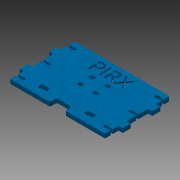
# Autodesk Inventor part: czesc5
Saved by Autodesk Inventor 2013 (Build 170138000, 138)
## iProperties
Created: 2014-01-17
Part Number: czesc5
Material: Generic
Document SubType Name: Modeling
Designer: dzban
Density: 1 g/cm^3
Author: dzban
Autodesk Inventor part; units mm, degrees
ref_plane "YZ Plane" through (0, 0, 0) normal (1, 0, 0) x (0, 1, 0)
ref_plane "XZ Plane" through (0, 0, 0) normal (0, 1, 0) x (-1, 0, 0)
ref_plane "XY Plane" through (0, 0, 0) normal (0, 0, 1) x (1, 0, 0)
sketch "Sketch1" plane through (0, 0, 0) normal (0, 0, 1) x (1, 0, 0)
  line L0 (24.6928, -26.0637) -> (24.6928, -36.0637)
  line L1 (24.6928, -36.0637) -> (83.1928, -36.0637)
  line L2 (83.1928, -36.0637) -> (83.1928, -27.5637)
  line L3 (83.1928, -27.5637) -> (76.1894, -27.5637)
  line L4 (76.1894, -27.5637) -> (76.1894, -28.8137)
  line L5 (76.1894, -28.8137) -> (74.3894, -28.8137)
  line L6 (74.3894, -28.8137) -> (74.3894, -27.5637)
  line L7 (74.3894, -27.5637) -> (71.3894, -27.5637)
  line L8 (71.3894, -27.5637) -> (71.3894, -24.5637)
  line L9 (71.3894, -24.5637) -> (74.3894, -24.5637)
  line L10 (74.3894, -24.5637) -> (74.3894, -23.3137)
  line L11 (74.3894, -23.3137) -> (76.1894, -23.3137)
  line L12 (76.1894, -23.3137) -> (76.1894, -24.5637)
  line L13 (76.1894, -24.5637) -> (83.1928, -24.5637)
  line L14 (83.1928, -24.5637) -> (83.1928, -16.1637)
  line L15 (83.1928, -16.1637) -> (89.1928, -16.0637)
  line L16 (89.1928, -16.0637) -> (89.1928, -4.2637)
  line L17 (89.1928, -4.2637) -> (83.1928, -4.1637)
  line L18 (83.1928, -4.1637) -> (83.1928, 9.9363)
  line L19 (83.1928, 9.9363) -> (76.1894, 9.9363)
  line L20 (76.1894, 9.9363) -> (76.1894, 8.6863)
  line L21 (76.1894, 8.6863) -> (74.3894, 8.6863)
  line L22 (74.3894, 8.6863) -> (74.3894, 9.9363)
  line L23 (74.3894, 9.9363) -> (71.3894, 9.9363)
  line L24 (71.3894, 9.9363) -> (71.3894, 12.9363)
  line L25 (71.3894, 12.9363) -> (74.3894, 12.9363)
  line L26 (74.3894, 12.9363) -> (74.3894, 14.1863)
  line L27 (74.3894, 14.1863) -> (76.1894, 14.1863)
  line L28 (76.1894, 14.1863) -> (76.1894, 12.9363)
  line L29 (76.1894, 12.9363) -> (83.1928, 12.9363)
  line L30 (83.1928, 12.9363) -> (83.1928, 27.0363)
  line L31 (83.1928, 27.0363) -> (89.1928, 27.1363)
  line L32 (89.1928, 27.1363) -> (89.1928, 38.9363)
  line L33 (89.1928, 38.9363) -> (83.1928, 39.0363)
  line L34 (83.1928, 39.0363) -> (83.1928, 47.4363)
  line L35 (83.1928, 47.4363) -> (76.1894, 47.4363)
  line L36 (76.1894, 47.4363) -> (76.1894, 46.1863)
  line L37 (76.1894, 46.1863) -> (74.3894, 46.1863)
  line L38 (74.3894, 46.1863) -> (74.3894, 47.4363)
  line L39 (74.3894, 47.4363) -> (71.3894, 47.4363)
  line L40 (71.3894, 47.4363) -> (71.3894, 50.4363)
  line L41 (71.3894, 50.4363) -> (74.3894, 50.4363)
  line L42 (74.3894, 50.4363) -> (74.3894, 51.6863)
  line L43 (74.3894, 51.6863) -> (76.1894, 51.6863)
  line L44 (76.1894, 51.6863) -> (76.1894, 50.4363)
  line L45 (76.1894, 50.4363) -> (83.1928, 50.4363)
  line L46 (83.1928, 50.4363) -> (83.1928, 52.9373)
  line L47 (83.1928, 55.937) -> (83.1928, 56.9363)
  arc A0 (83.1928, 56.9363) -> (81.1928, 58.9363) centre (81.1928, 56.9363) ccw
  line L48 (81.1928, 58.9363) -> (-53.8072, 58.9363)
  arc A1 (-53.8072, 58.9363) -> (-55.8072, 56.9363) centre (-53.8072, 56.9363) ccw
  line L49 (-55.8072, 56.9363) -> (-55.8072, 55.9363)
  line L50 (-55.8072, 52.9363) -> (-55.8072, 50.4363)
  line L51 (-55.8072, 50.4363) -> (-48.8072, 50.4363)
  line L52 (-48.8072, 50.4363) -> (-48.8072, 51.6863)
  line L53 (-48.8072, 51.6863) -> (-47.0072, 51.6863)
  line L54 (-47.0072, 51.6863) -> (-47.0072, 50.4363)
  line L55 (-47.0072, 50.4363) -> (-44.0716, 50.4363)
  line L56 (-44.0716, 50.4363) -> (-44.0716, 47.4363)
  line L57 (-44.0716, 47.4363) -> (-47.0072, 47.4363)
  line L58 (-47.0072, 47.4363) -> (-47.0072, 46.1863)
  line L59 (-47.0072, 46.1863) -> (-48.8072, 46.1863)
  line L60 (-48.8072, 46.1863) -> (-48.8072, 47.4363)
  line L61 (-48.8072, 47.4363) -> (-55.8072, 47.4363)
  line L62 (-55.8072, 47.4363) -> (-55.8072, 39.0363)
  line L63 (-55.8072, 39.0363) -> (-61.8072, 38.9363)
  line L64 (-61.8072, 38.9363) -> (-61.8072, 27.1363)
  line L65 (-61.8072, 27.1363) -> (-55.8072, 27.0363)
  line L66 (-55.8072, 27.0363) -> (-55.8072, 12.9363)
  line L67 (-55.8072, 12.9363) -> (-48.8072, 12.9363)
  line L68 (-48.8072, 12.9363) -> (-48.8072, 14.1863)
  line L69 (-48.8072, 14.1863) -> (-47.0072, 14.1863)
  line L70 (-47.0072, 14.1863) -> (-47.0072, 12.9363)
  line L71 (-47.0072, 12.9363) -> (-44.0716, 12.9363)
  line L72 (-44.0716, 12.9363) -> (-44.0716, 9.9363)
  line L73 (-44.0716, 9.9363) -> (-47.0072, 9.9363)
  line L74 (-47.0072, 9.9363) -> (-47.0072, 8.6863)
  line L75 (-47.0072, 8.6863) -> (-48.8072, 8.6863)
  line L76 (-48.8072, 8.6863) -> (-48.8072, 9.9363)
  line L77 (-48.8072, 9.9363) -> (-55.8072, 9.9363)
  line L78 (-55.8072, 9.9363) -> (-55.8072, -4.1637)
  line L79 (-55.8072, -4.1637) -> (-61.8072, -4.2637)
  line L80 (-61.8072, -4.2637) -> (-61.8072, -16.0637)
  line L81 (-61.8072, -16.0637) -> (-55.8072, -16.1637)
  line L82 (-55.8072, -16.1637) -> (-55.8072, -24.5637)
  line L83 (-55.8072, -24.5637) -> (-48.8072, -24.5637)
  line L84 (-48.8072, -24.5637) -> (-48.8072, -23.3137)
  line L85 (-48.8072, -23.3137) -> (-47.0072, -23.3137)
  line L86 (-47.0072, -23.3137) -> (-47.0072, -24.5637)
  line L87 (-47.0072, -24.5637) -> (-44.0716, -24.5637)
  line L88 (-44.0716, -24.5637) -> (-44.0716, -27.5637)
  line L89 (-44.0716, -27.5637) -> (-47.0072, -27.5637)
  line L90 (-47.0072, -27.5637) -> (-47.0072, -28.8137)
  line L91 (-47.0072, -28.8137) -> (-48.8072, -28.8137)
  line L92 (-48.8072, -28.8137) -> (-48.8072, -27.5637)
  line L93 (-48.8072, -27.5637) -> (-55.8072, -27.5637)
  line L94 (-55.8072, -27.5637) -> (-55.8072, -36.0637)
  line L95 (-55.8072, -36.0637) -> (2.6928, -36.0637)
  line L96 (2.6928, -36.0637) -> (2.6928, -26.0637)
  line L97 (2.6928, -26.0637) -> (24.6928, -26.0637)
  line L98 (53.2575, -19.0636) -> (53.2575, -25.4636)
  line L99 (53.2575, -25.4636) -> (41.4575, -25.4636)
  line L100 (41.4575, -25.4636) -> (41.4575, -19.0636)
  line L101 (41.4575, -19.0636) -> (53.2575, -19.0636)
  line L102 (-13.9425, -19.0636) -> (-13.9425, -25.4636)
  line L103 (-13.9425, -25.4636) -> (-25.7425, -25.4636)
  line L104 (-25.7425, -25.4636) -> (-25.7425, -19.0636)
  line L105 (-25.7425, -19.0636) -> (-13.9425, -19.0636)
  line L106 (5.6928, 6.2364) -> (-0.7072, 6.2364)
  line L107 (-0.7072, 6.2364) -> (-0.7072, 11.2364)
  line L108 (-0.7072, 11.2364) -> (5.6928, 11.2364)
  line L109 (5.6928, 11.2364) -> (5.6928, 6.2364)
  line L110 (28.0928, 6.2364) -> (21.6928, 6.2364)
  line L111 (21.6928, 6.2364) -> (21.6928, 11.2364)
  line L112 (21.6928, 11.2364) -> (28.0928, 11.2364)
  line L113 (28.0928, 11.2364) -> (28.0928, 6.2364)
  line L114 (28.0928, 23.8364) -> (21.6928, 23.8364)
  line L115 (21.6928, 23.8364) -> (21.6928, 28.8364)
  line L116 (21.6928, 28.8364) -> (28.0928, 28.8364)
  line L117 (28.0928, 28.8364) -> (28.0928, 23.8364)
  line L118 (5.6928, 28.8364) -> (5.6928, 23.8364)
  line L119 (5.6928, 23.8364) -> (-0.7072, 23.8364)
  line L120 (-0.7072, 23.8364) -> (-0.7072, 28.8364)
  line L121 (-0.7072, 28.8364) -> (5.6928, 28.8364)
  line L122 (-55.8072, 52.9363) -> (-55.8072, 55.9363)
  line L123 (83.1928, 52.9373) -> (83.1928, 55.937)
  point P0 (0, 0)
  dimension "d0" = 58.9363
  dimension "d2" = 139
  dimension "d3" = 95
  dimension "d4" = 55.8072
  dimension "d5" = 6
  dimension "d6" = 2
  dimension "d7" = 12
  dimension "d8" = 12
  dimension "d9" = 11.7356
  dimension "d10" = 2.9356
  dimension "d11" = 1.8
  dimension "d12" = 3
  dimension "d13" = 1.25
  dimension "d14" = 1.25
  dimension "d15" = 8.5
  dimension "d16" = 3
  dimension "d17" = 1.25
  dimension "d18" = 1.25
  dimension "d19" = 8.5
  dimension "d20" = 19.9
  dimension "d21" = 0.1
  dimension "d22" = 11.8
  dimension "d23" = 46
  dimension "d24" = 3
  dimension "d25" = 1.25
  dimension "d26" = 1.25
  dimension "d27" = 19.9
  dimension "d28" = 6.4
  dimension "d29" = 5
  dimension "d30" = 6.4
  dimension "d31" = 5
  dimension "d32" = 12.6
  dimension "d33" = 16
  dimension "d34" = 30.1
  dimension "d35" = 55.1
  dimension "d36" = 11.8033
  dimension "d37" = 3
  dimension "d38" = 1.8
  dimension "d39" = 6
  dimension "d40" = 22
  dimension "d41" = 10
  dimension "d42" = 58.5
  constraints: 248 end point, 88 parallel, 65 collinear, 24 perpendicular, 16 tangent, 4 horizontal alignment, 4 point on circle, 2 centre point, 1 equal radius, 1 horizontal
  measures "d0" distance from line of L48 point (0, 0)
  measures "d2" distance between parallel lines of L47 L49
  measures "d3" distance between parallel lines of L48 L95
  measures "d4" distance from line of L49 point (0, 0)
  measures "d5" distance between parallel lines of L94 L80
  measures "d6" radius of A1
  measures "d7" distance of L62.end L65.end
  measures "d8" distance of L78.end L81.end
  measures "d9" distance between parallel lines of L50 L56
  measures "d10" distance between parallel lines of L56 L54
  measures "d11" distance between parallel lines of L54 L52
  measures "d12" distance between parallel lines of L51 L61
  measures "d13" distance between parallel lines of L53 L51
  measures "d14" distance from line of L57 L58.end
  measures "d15" distance between parallel lines of L48 L51
  measures "d16" distance between parallel lines of L83 L93
  measures "d17" distance between parallel lines of L89 L91
  measures "d18" distance between parallel lines of L85 L87
  measures "d19" distance between parallel lines of L93 L95
  measures "d20" distance from line of L48 L62.end
  measures "d21" vertical distance of L62.end L63.end
  measures "d22" distance of L63.end L64.end
  measures "d23" distance between parallel lines of L77 L95
  measures "d24" distance between parallel lines of L67 L77
  measures "d25" distance between parallel lines of L73 L75
  measures "d26" distance between parallel lines of L71 L69
  measures "d27" distance from line of L81.end L95
  measures "d28" distance between parallel lines of L118 L120
  measures "d29" distance between parallel lines of L121 L119
  measures "d30" distance between parallel lines of L117 L115
  measures "d31" distance between parallel lines of L108 L106
  measures "d32" distance between parallel lines of L119 L108
  measures "d33" distance between parallel lines of L115 L118
  measures "d34" distance between parallel lines of L48 L121
  measures "d35" distance between parallel lines of L120 L66
  measures "d36" distance between parallel lines of L46 L40
  measures "d37" distance between parallel lines of L42 L40
  measures "d38" distance between parallel lines of L44 L42
  measures "d39" distance from line of L47.start L32
  measures "d40" distance between parallel lines of L0 L96
  measures "d41" distance between parallel lines of L97 L1
  measures "d42" distance between parallel lines of L96 L94
extrude "Extrusion1" add sketch "Sketch1" along normal blind 6
fillet "Fillet1" radius 2 4 edges at (2.6928, -36.0637, 3) (2.6928, -26.0637, 3) (24.6928, -26.0637, 3) (24.6928, -36.0637, 3)
sketch "Sketch9" plane through (0, 0, 6) normal (0, 0, 1) x (1, 0, 0)
  line L0 (-15.0286, 52.3696) -> (-4.2568, 52.3696) construction
  line L1 (-4.2568, 52.3696) -> (-4.2568, 48.8696) construction
  line L2 (-4.2568, 48.8696) -> (-15.0286, 48.8696) construction
  line L3 (-15.0286, 48.8696) -> (-15.0286, 52.3696) construction
  line L4 (-10.157, 41.1104) -> (-10.157, 34.3696)
  line L5 (-10.157, 34.3696) -> (-12.5855, 34.3696)
  line L6 (-12.5855, 34.3696) -> (-12.5855, 52.3696)
  line L7 (-12.5855, 52.3696) -> (-7.2723, 52.3696)
  spline S0 degree 2 poles (-7.2723, 52.3696) (-5.565, 52.3696) (-3.0483, 51.5748) (-1.3851, 50.1178) (-0.5757, 48.0572) (-0.5757, 46.7915) knots 0 0 0 1 2 3 4 4 4
  spline S1 degree 2 poles (-0.5757, 46.7915) (-0.5757, 45.5405) (-1.4587, 43.4505) (-3.1513, 41.9493) (-5.6533, 41.1104) (-7.2723, 41.1104) knots 0 0 0 1 2 3 4 4 4
  line L8 (-7.2723, 41.1104) -> (-10.157, 41.1104)
  line L9 (-10.157, 43.0384) -> (-7.2723, 43.0384)
  spline S2 degree 2 poles (-7.2723, 43.0384) (-6.242, 43.0384) (-4.6525, 43.5977) (-3.5634, 44.5838) (-3.0188, 45.9673) (-3.0188, 46.7915) knots 0 0 0 1 2 3 4 4 4
  spline S3 degree 2 poles (-3.0188, 46.7915) (-3.0188, 48.5135) (-5.1382, 50.4416) (-7.2723, 50.4416) knots 0 0 0 1 2 2 2
  line L10 (-7.2723, 50.4416) -> (-10.157, 50.4416)
  line L11 (-10.157, 50.4416) -> (-10.157, 43.0384)
  line L12 (5.3998, 34.3696) -> (2.9566, 34.3696)
  line L13 (2.9566, 34.3696) -> (2.9566, 52.3696)
  line L14 (2.9566, 52.3696) -> (5.3998, 52.3696)
  line L15 (5.3998, 52.3696) -> (5.3998, 34.3696)
  line L16 (12.906, 41.8904) -> (12.906, 34.3696)
  line L17 (12.906, 34.3696) -> (10.4775, 34.3696)
  line L18 (10.4775, 34.3696) -> (10.4775, 52.3696)
  line L19 (10.4775, 52.3696) -> (15.5552, 52.3696)
  spline S4 degree 2 poles (15.5552, 52.3696) (17.2625, 52.3696) (19.7498, 51.6779) (21.3687, 50.368) (22.1488, 48.5282) (22.1488, 47.3802) knots 0 0 0 1 2 3 4 4 4
  spline S5 degree 2 poles (22.1488, 47.3802) (22.1488, 46.4383) (21.5454, 44.7752) (20.3974, 43.4653) (18.7637, 42.5233) (17.7187, 42.2878) knots 0 0 0 1 2 3 4 4 4
  spline S6 degree 2 poles (17.7187, 42.2878) (18.175, 42.0229) (18.5282, 41.5225) knots 0 0 0 1 1 1
  line L20 (18.5282, 41.5225) -> (23.7678, 34.3696)
  line L21 (23.7678, 34.3696) -> (21.619, 34.3696)
  spline S7 degree 2 poles (21.619, 34.3696) (20.9419, 34.3696) (20.6329, 34.8847) knots 0 0 0 1 1 1
  line L22 (20.6329, 34.8847) -> (15.9673, 41.3312)
  spline S8 degree 2 poles (15.9673, 41.3312) (15.7465, 41.6255) (15.2461, 41.8904) (14.7457, 41.8904) knots 0 0 0 1 2 2 2
  line L23 (14.7457, 41.8904) -> (12.906, 41.8904)
  line L24 (12.906, 43.6566) -> (15.4521, 43.6566)
  spline S9 degree 2 poles (15.4521, 43.6566) (16.5118, 43.6566) (18.1308, 44.1717) (19.2346, 45.1137) (19.7792, 46.4088) (19.7792, 47.2036) knots 0 0 0 1 2 3 4 4 4
  spline S10 degree 2 poles (19.7792, 47.2036) (19.7792, 48.8079) (17.6598, 50.4416) (15.5699, 50.4416) knots 0 0 0 1 2 2 2
  line L25 (15.5699, 50.4416) -> (12.906, 50.4416)
  line L26 (12.906, 50.4416) -> (12.906, 43.6566)
  line L27 (30.5822, 43.6124) -> (24.6361, 52.3696)
  line L28 (24.6361, 52.3696) -> (27.0646, 52.3696)
  spline S11 degree 2 poles (27.0646, 52.3696) (27.3295, 52.3696) (27.5797, 52.193) (27.6827, 52.0311) knots 0 0 0 1 2 2 2
  line L29 (27.6827, 52.0311) -> (32.3777, 44.8193)
  spline S12 degree 2 poles (32.3777, 44.8193) (32.466, 45.0842) (32.6427, 45.3933) knots 0 0 0 1 1 1
  line L30 (32.6427, 45.3933) -> (37.0728, 51.9869)
  spline S13 degree 2 poles (37.0728, 51.9869) (37.1905, 52.1488) (37.4554, 52.3696) (37.632, 52.3696) knots 0 0 0 1 2 2 2
  line L31 (37.632, 52.3696) -> (39.9575, 52.3696)
  line L32 (39.9575, 52.3696) -> (33.9967, 43.7302)
  line L33 (33.9967, 43.7302) -> (40.1635, 34.3696)
  line L34 (40.1635, 34.3696) -> (37.7498, 34.3696)
  spline S14 degree 2 poles (37.7498, 34.3696) (37.4701, 34.3696) (37.1611, 34.664) (37.058, 34.8406) knots 0 0 0 1 2 2 2
  line L35 (37.058, 34.8406) -> (32.2306, 42.3909)
  spline S15 degree 2 poles (32.2306, 42.3909) (32.1423, 42.1259) (32.0098, 41.8757) knots 0 0 0 1 1 1
  line L36 (32.0098, 41.8757) -> (27.3148, 34.8406)
  spline S16 degree 2 poles (27.3148, 34.8406) (27.197, 34.664) (26.9174, 34.3696) (26.6525, 34.3696) knots 0 0 0 1 2 2 2
  line L37 (26.6525, 34.3696) -> (24.3859, 34.3696)
  line L38 (24.3859, 34.3696) -> (30.5822, 43.6124)
  point P0 (0, 0)
  constraints: 2 other
extrude "Extrusion9" cut sketch "Sketch9" against normal blind 10
sketch "Sketch10" plane through (0, 0, 6) normal (0, 0, 1) x (1, 0, 0)
  line L0 (-14.2237, 48.1332) -> (-8.3029, 48.1332)
  line L1 (-8.3029, 48.1332) -> (-8.3029, 45.8332)
  line L2 (-8.3029, 45.8332) -> (-14.2237, 45.8332)
  line L3 (-14.2237, 45.8332) -> (-14.2237, 48.1332)
  line L4 (9.4512, 48.1332) -> (15.0431, 48.1332)
  line L5 (15.0431, 48.1332) -> (15.0431, 45.8332)
  line L6 (15.0431, 45.8332) -> (9.4512, 45.8332)
  line L7 (9.4512, 45.8332) -> (9.4512, 48.1332)
  point P0 (0, 0)
  dimension "d79" = 2.3
  constraints: 16 end point, 4 parallel, 2 collinear, 2 horizontal, 2 perpendicular
  measures "d79" distance between parallel lines of L0 L2
extrude "Extrusion10" add sketch "Sketch10" against normal blind 6
sketch "Sketch5" plane through (0, 0, 6) normal (0, 0, 1) x (1, 0, 0)
  line L0 (26.6928, -36.0637) -> (83.1928, -36.0637) projected
  line L1 (5.6928, 6.2364) -> (-0.7072, 6.2364) projected
  line L2 (-13.9467, 32.2205) -> (46.2491, 32.2205)
  point P0 (0, 0)
  constraints: 2 end point, 2 parallel, 1 horizontal
sketch "Sketch6" plane through (0, 0, 6) normal (0, 0, 1) x (1, 0, 0)
  line L0 (-5.754, 45.1214) -> (-13.9983, 45.1214)
  line L1 (-13.9983, 45.1214) -> (-13.9983, 43.2496)
  line L2 (-13.9983, 43.2496) -> (-5.754, 43.2496)
  line L3 (-5.754, 43.2496) -> (-5.754, 45.1214)
  point P0 (0, 0)
  constraints: 8 end point, 2 parallel, 1 horizontal, 1 perpendicular
sketch "Sketch3" plane through (0, 0, 6) normal (0, 0, 1) x (1, 0, 0)
  line L0 (81.1928, 58.9363) -> (-53.8072, 58.9363) projected
  line L1 (-55.8072, 56.9363) -> (-55.8072, 50.4363) projected
  circle A0 centre (13.6928, 145.3363) radius 101.6
  point P0 (0, 0)
  dimension "d49" = 69.5
  dimension "d50" = 86.4
  dimension "d51" = 203.2
  constraints: 1 centre point
  measures "d49" distance from line of L1 A0.centre
  measures "d50" distance from line of A0.centre L0
  measures "d51" diameter of A0
body "Solid1"
